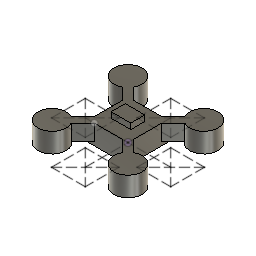
abxy-pcb-jig v1 (Autodesk Fusion 360 design; units mm, degrees)
Autodesk Fusion 360 part; units mm, degrees
sketch "Sketch1" plane through (0, 0, 0) normal (0, 0, 1) x (1, 0, 0)
  line L0 (-3, 10.6) -> (3, 10.6) construction
  line L1 (3, 10.6) -> (3, 4.6) construction
  line L2 (3, 4.6) -> (-3, 4.6) construction
  line L3 (-3, 4.6) -> (-3, 10.6) construction
  line L4 (0, -7.6) -> (0, 7.6) construction
  line L5 (0, 0) -> (-6, 0) construction
  line L6 (-3, 10.6) -> (3, 4.6) construction
  line L7 (3, 10.6) -> (-3, 4.6) construction
  line L8 (-3, -4.6) -> (3, -4.6) construction
  line L9 (3, -4.6) -> (3, -10.6) construction
  line L10 (3, -10.6) -> (-3, -10.6) construction
  line L11 (-3, -10.6) -> (-3, -4.6) construction
  line L12 (4.6, 3) -> (10.6, 3) construction
  line L13 (10.6, 3) -> (10.6, -3) construction
  line L14 (10.6, -3) -> (4.6, -3) construction
  line L15 (4.6, -3) -> (4.6, 3) construction
  line L16 (-10.6, 3) -> (-4.6, 3) construction
  line L17 (-4.6, 3) -> (-4.6, -3) construction
  line L18 (-4.6, -3) -> (-10.6, -3) construction
  line L19 (-10.6, -3) -> (-10.6, 3) construction
  line L20 (-7.6, 0) -> (7.6, 0) construction
  line L21 (-10.6, 3) -> (-4.6, -3) construction
  line L22 (-4.6, 3) -> (-10.6, -3) construction
  line L23 (-3, -10.6) -> (3, -4.6) construction
  line L24 (-3, -4.6) -> (3, -10.6) construction
  line L25 (4.6, 3) -> (10.6, -3) construction
  line L26 (10.6, 3) -> (4.6, -3) construction
  dimension "d1" = 6
  dimension "d3" = 15.2
  constraint horizontal L0
  constraint vertical L1
  constraint horizontal L2
  constraint vertical L3
  constraint perpendicular L2 L4
  constraint coincident L5.start origin
  constraint perpendicular L4 L5
  constraint symmetric L4.start L4.end L5
  constraint coincident L5.start L4
  constraint coincident L4.end L6
  constraint coincident L4.end L7
  constraint equal L0 L3
  constraint horizontal L8
  constraint vertical L9
  constraint horizontal L10
  constraint vertical L11
  constraint horizontal L12
  constraint vertical L13
  constraint horizontal L14
  constraint vertical L15
  constraint horizontal L16
  constraint vertical L17
  constraint horizontal L18
  constraint vertical L19
  constraint perpendicular L17 L20
  constraint symmetric L4 L20.start L20.end
  constraint equal L4 L20
  constraint equal L12 L15
  constraint equal L8 L15
  constraint equal L8 L11
  constraint equal L11 L16
  constraint equal L16 L19
  constraint equal L3 L19
  constraint coincident L20.end L26
  constraint coincident L20.end L25
  constraint coincident L20.start L22
  constraint coincident L20.start L21
  constraint coincident L4.start L24
  constraint coincident L4.start L23
  constraint coincident L5.start L20
  measures "d1" distance of L0.start L2.end
  measures "d3" distance of L4.start L4.end
sketch "Sketch5" plane through (0, 0, 0) normal (0, 0, 1) x (1, 0, 0)
  line L0 (-3.5, 3.5) -> (3.5, 3.5)
  line L1 (3.5, 3.5) -> (3.5, -3.5)
  line L2 (3.5, -3.5) -> (-3.5, -3.5)
  line L3 (-3.5, -3.5) -> (-3.5, 3.5)
  line L4 (-3.5, 3.5) -> (3.5, -3.5) construction
  line L5 (3.5, 3.5) -> (-3.5, -3.5) construction
  dimension "d11" = 7
  constraint horizontal L0
  constraint vertical L1
  constraint horizontal L2
  constraint vertical L3
  constraint perpendicular L4 L5
  constraint coincident L5 origin
  constraint coincident L4 origin
  measures "d11" distance of L0.start L0.end
extrude "Extrude4" add sketch "Sketch5" along normal blind 3.5 makes body 1
sketch "Sketch6" plane through (0, 0, 0) normal (0, 0, 1) x (1, 0, 0)
  circle A0 centre (-6.75, 6.75) radius 2.5
  circle A1 centre (6.75, 6.75) radius 2.5
  circle A2 centre (6.75, -6.75) radius 2.5
  circle A3 centre (-6.75, -6.75) radius 2.5
  line L0 (-6.75, 6.75) -> (6.75, 6.75) construction
  line L1 (6.75, 6.75) -> (6.75, -6.75) construction
  line L2 (6.75, -6.75) -> (-6.75, -6.75) construction
  line L3 (-6.75, -6.75) -> (-6.75, 6.75) construction
  line L4 (6.75, 6.75) -> (-6.75, -6.75) construction
  line L5 (-6.75, 6.75) -> (6.75, -6.75) construction
  point P0 (-7.6, 0)
  point P1 (7.6, 0)
  point P2 (0, 7.6)
  point P3 (0, -7.6)
  dimension "d14" = 5
  dimension "d15" = 13.5
  constraint equal A0 A1
  constraint equal A1 A2
  constraint equal A2 A3
  constraint horizontal L0
  constraint vertical L1
  constraint horizontal L2
  constraint vertical L3
  constraint coincident A2.centre L1.end
  constraint coincident A0.centre L0.start
  constraint coincident A1.centre L0.end
  constraint coincident A3.centre L2.end
  constraint equal L0 L1
  constraint coincident origin L5
  constraint coincident origin L4
  measures "d14" diameter of A0
  measures "d15" distance of A1.centre A2.centre
extrude "Extrude5" add sketch "Sketch6" along normal blind 3.5 separate body makes body 2 at (9.2376, 6.5011, 2.3333) makes body 3 at (9.2376, -6.9989, 2.3333) makes body 4 at (-4.2624, 6.5011, 2.3333) makes body 5 at (-4.2624, -6.9989, 2.3333)
ref_plane "WorkPlane1" through (0, 0, 0.75) normal (0, 0, 1) x (1, 0, 0)
sketch "Sketch7" plane through (0, 0, 0.75) normal (0, 0, 1) x (1, 0, 0)
  line L0 (-5.594, 4.5333) -> (4.5333, -5.594)
  line L1 (4.5333, -5.594) -> (5.594, -4.5333)
  line L2 (5.594, -4.5333) -> (-4.5333, 5.594)
  line L3 (-4.5333, 5.594) -> (-5.594, 4.5333)
  line L4 (5.594, 4.5333) -> (4.5333, 5.594)
  line L5 (4.5333, 5.594) -> (-5.594, -4.5333)
  line L6 (-5.594, -4.5333) -> (-4.5333, -5.594)
  line L7 (-4.5333, -5.594) -> (5.594, 4.5333)
  line L8 (-7.6, 0) -> (7.6, 0)
  line L9 (-1.0607, 0) -> (1.0607, 0) construction
  line L10 (0, -7.6) -> (0, 7.6) construction
  circle A0 centre (6.75, 6.75) radius 2.5 construction
  circle A1 centre (-6.75, 6.75) radius 2.5 construction
  circle A2 centre (-6.75, -6.75) radius 2.5 construction
  circle A3 centre (6.75, -6.75) radius 2.5 construction
  dimension "d18" = 45
  dimension "d19" = 1.5
  constraint perpendicular L0 L1
  constraint parallel L0 L2
  constraint parallel L1 L3
  constraint perpendicular L4 L5
  constraint parallel L4 L6
  constraint parallel L5 L7
  constraint perpendicular L3 L4
  constraint equal L3 L4
  constraint coincident L8 L9.start
  constraint coincident L0 L9.start
  constraint coincident L8 L9.end
  constraint coincident L2 L9.end
  constraint coincident L5 L9.start
  constraint symmetric L9.start L9.end L10
  constraint coincident L2.end A1
  constraint coincident L4.end A0
  constraint coincident L5.end A2
  constraint coincident L1.end A3
  measures "d18" angle of L5 L8
  measures "d19" distance of L0.start L2.end
extrude "Extrude6" add sketch "Sketch7" along normal up to surface (2.75 mm away) contours L0 L2 L3 L5 | L0 L5 L6 L7 | L0 L1 L2 L7 | L2 L4 L5 L7 bodies 1 2 3 4 5
sketch "Sketch9" plane through (0, 0, 0) normal (0, 0, 1) x (1, 0, 0)
  circle A0 centre (0, 0) radius 0.675
  dimension "d23" = 1.35
  constraint coincident A0.centre origin
  measures "d23" diameter of A0
extrude "Extrude7" cut sketch "Sketch9" along normal blind 3 bodies 1
sketch "Sketch10" plane through (0, 0, 3.5) normal (0, 0, 1) x (-1, 0, 0)
  arc A0 (4.5333, -5.594) -> (5.594, -4.5333) centre (6.75, -6.75) ccw
  line L0 (5.594, -4.5333) -> (3.5, -2.4393)
  line L1 (3.5, -2.4393) -> (3.5, 2.4393)
  line L2 (3.5, 2.4393) -> (5.594, 4.5333)
  arc A1 (5.594, 4.5333) -> (4.5333, 5.594) centre (6.75, 6.75) ccw
  line L3 (4.5333, 5.594) -> (2.4393, 3.5)
  line L4 (2.4393, 3.5) -> (-2.4393, 3.5)
  line L5 (-2.4393, 3.5) -> (-4.5333, 5.594)
  arc A2 (-4.5333, 5.594) -> (-5.594, 4.5333) centre (-6.75, 6.75) ccw
  line L6 (-5.594, 4.5333) -> (-3.5, 2.4393)
  line L7 (-3.5, 2.4393) -> (-3.5, -2.4393)
  line L8 (-3.5, -2.4393) -> (-5.594, -4.5333)
  arc A3 (-5.594, -4.5333) -> (-4.5333, -5.594) centre (-6.75, -6.75) ccw
  line L9 (-4.5333, -5.594) -> (-2.4393, -3.5)
  line L10 (-2.4393, -3.5) -> (2.4393, -3.5)
  line L11 (2.4393, -3.5) -> (4.5333, -5.594)
  line L12 (1.75, -1.25) -> (-1.75, -1.25)
  line L13 (-1.75, -1.25) -> (-1.75, 1.25)
  line L14 (-1.75, 1.25) -> (1.75, 1.25)
  line L15 (1.75, 1.25) -> (1.75, -1.25)
  line L16 (1.75, -1.25) -> (-1.75, 1.25) construction
  line L17 (-1.75, -1.25) -> (1.75, 1.25) construction
  dimension "d26" = 3.5
  dimension "d27" = 2.5
  constraint horizontal L12
  constraint vertical L13
  constraint horizontal L14
  constraint vertical L15
  constraint coincident origin L17
  constraint coincident origin L16
  measures "d26" distance of L12.start L12.end
  measures "d27" distance of L12.end L13.end
extrude "Extrude8" add sketch "Sketch10" along normal blind 1 contours L12 L13 L14 L15 bodies 1
